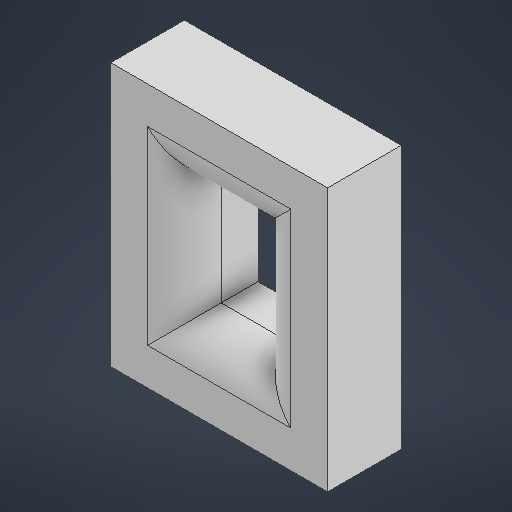
# Autodesk Inventor part: Motor Fitting Test 2
Saved by Autodesk Inventor 2026.1 (Build 301233000, 233)
## iProperties
Created: 2025-11-04
Part Number: Motor Fitting Test 2
Material: Generic
Document SubType Name: Modeling
Designer: uu-112
Density: 1 g/cm^3
Appearance: Default
Author: uu-112
Autodesk Inventor part; units mm, degrees
ref_plane "YZ Plane" through (0, 0, 0) normal (1, 0, 0) x (0, 1, 0)
ref_plane "XZ Plane" through (0, 0, 0) normal (0, 1, 0) x (-1, 0, 0)
ref_plane "XY Plane" through (0, 0, 0) normal (0, 0, 1) x (1, 0, 0)
sketch "Sketch1" plane through (0, 0, 0) normal (0, 0, 1) x (1, 0, 0)
  line L0 (-1.5, 2.5) -> (1.5, 2.5)
  line L1 (1.5, 2.5) -> (1.5, -2.5)
  line L2 (1.5, -2.5) -> (-1.5, -2.5)
  line L3 (-1.5, -2.5) -> (-1.5, 2.5)
  line L4 (-1.5, 2.5) -> (1.5, -2.5) construction
  line L5 (1.5, 2.5) -> (-1.5, -2.5) construction
  line L6 (4.675, 5.675) -> (-4.675, 5.675)
  line L7 (-4.675, 5.675) -> (-4.675, -5.675)
  line L8 (-4.675, -5.675) -> (4.675, -5.675)
  line L9 (4.675, -5.675) -> (4.675, 5.675)
  point P0 (0, 0)
  dimension "d0" = 3
  dimension "d1" = 5
  dimension "d2" = 3.175
  constraints: 20 end point, 4 parallel, 2 midpoint, 2 perpendicular, 1 horizontal, 3 other
  measures "d0" distance of L1.end L2.end
  measures "d1" distance of L0.end L1.end
  measures "d2" distance between parallel lines of L0 L6
extrude "Extrusion1" add sketch "Sketch1" along normal mid plane 3.175
fillet "Fillet1" radius 1.5875 2 edges at (0, 2.5, 1.5875) (0, -2.5, 1.5875)
fillet "Fillet2" radius 1.5875 2 edges at (-1.5, 0, 1.5875) (1.5, 0, 1.5875)
body "Solid1"
